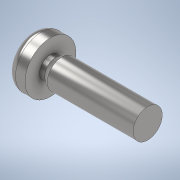
# Autodesk Inventor part: 13-螺钉
Saved by Autodesk Inventor 2022 (Build 260153000, 153)
## iProperties
Created: 2023-01-09
Part Number: 13-螺钉
Material: 不锈钢
Document SubType Name: Modeling
Designer: Lzy18
Density: 8 g/cm^3
Appearance: 半抛光
Author: Lzy18
Autodesk Inventor part; units mm, degrees
ref_plane "YZ Plane" through (0, 0, 0) normal (1, 0, 0) x (0, 1, 0)
ref_plane "XZ Plane" through (0, 0, 0) normal (0, 1, 0) x (-1, 0, 0)
ref_plane "XY Plane" through (0, 0, 0) normal (0, 0, 1) x (1, 0, 0)
sketch "草图1" plane through (0, 0, 0) normal (0, 0, 1) x (1, 0, 0)
  line L0 (0, 0) -> (1.4, 0)
  line L1 (1.4, -3) -> (0, -3)
  line L2 (0, 0) -> (-3, 0)
  line L3 (-3, -7) -> (0, -7)
  line L4 (0, -7) -> (0, -3)
  line L5 (-5, -4.6) -> (-5, -1)
  line L6 (-5, -1) -> (-3, -1)
  line L7 (-3, -6.9664) -> (-3, -7)
  arc A0 (-5, -4.6) -> (-2.6, -7) centre (-2.6, -4.6) ccw
  line L8 (1.4, -3) -> (3.1321, -4)
  line L9 (-3, 0) -> (-3, -1)
  line L10 (-3, -6.9664) -> (-3, -7)
  line L11 (1.4, 0) -> (26.7321, 0)
  line L12 (26.7321, 0) -> (26.7321, -4)
  line L13 (26.7321, -4) -> (3.1321, -4)
  dimension "d0" = 1.4
  dimension "d1" = 3
  dimension "d2" = 3
  dimension "d4" = 2
  dimension "d6" = 4.8
  dimension "d7" = 30
  dimension "d9" = 23.6
  dimension "d10" = 4
  constraints: 28 end point, 6 parallel, 3 horizontal, 3 perpendicular, 3 point on circle, 1 centre point, 1 point on line, 1 tangent
  measures "d0" distance of L1.end L1.start
  measures "d1" distance of L1.start L0.end
  measures "d2" distance of L3.end L3.start
  measures "d4" distance of L5.end L6.end
  measures "d6" diameter of A0
  measures "d7" angle of L0 L8
  measures "d9" distance of L8.end L12.end
  measures "d10" distance of L11.end L12.end
revolve "旋转1" add sketch "草图1" angle 360 about axis through (1.4, 0, 0) along (1, 0, 0) contours L0 L11 L12 L13 L8 L1 L4 L3 A0 L5 L6 L9 L2
